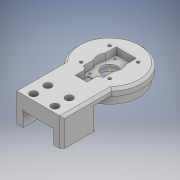
# Autodesk Inventor part: base_top
Saved by Autodesk Inventor 2017 (Build 210142000, 142)
## iProperties
Created: 2021-02-25
Part Number: base_top
Material: Generic
Document SubType Name: Modeling
Designer: paulg
Density: 1 g/cm^3
Appearance: Default
Author: paulg
Autodesk Inventor part; units mm, degrees
ref_plane "YZ Plane" through (0, 0, 0) normal (1, 0, 0) x (0, 1, 0)
ref_plane "XZ Plane" through (0, 0, 0) normal (0, 1, 0) x (-1, 0, 0)
ref_plane "XY Plane" through (0, 0, 0) normal (0, 0, 1) x (1, 0, 0)
sketch "Sketch1" plane through (0, 0, 0) normal (0, 0, 1) x (1, 0, 0)
  circle A0 centre (0, 0) radius 6.5
  circle A1 centre (0, 0) radius 25
  dimension "d0" = 50
  dimension "d1" = 13
  constraints: 2 centre point, 2 coincident
  measures "d0" diameter of A1
  measures "d1" diameter of A0
extrude "Extrusion1" add sketch "Sketch1" along normal blind 7
sketch "Sketch2" plane through (0, 0, 7) normal (0, 0, 1) x (1, 0, 0)
  circle A0 centre (0, 0) radius 6.5 projected
  circle A1 centre (0, 0) radius 25 projected
  circle A2 centre (0, 0) radius 27
  dimension "d4" = 2
  constraints: 1 centre point
  measures "d4" radial gap between concentric circles of A1 A2
extrude "Extrusion2" add sketch "Sketch2" along normal blind 1 contours A1 | A2
sketch "Sketch3" plane through (0, 0, 8) normal (0, 0, 1) x (1, 0, 0)
  circle A0 centre (0, 0) radius 6.5 projected
  circle A1 centre (0, 0) radius 27 projected
  line L0 (0, 0) -> (0, -39.0692) construction
  circle A2 centre (0, 0) radius 27 projected
  line L1 (20, -60) -> (-20, -60)
  line L2 (-20, -60) -> (-20, -18.1384)
  line L3 (-20, -18.1384) -> (20, -18.1384) construction
  line L4 (20, -18.1384) -> (20, -60)
  line L5 (20, -60) -> (-20, -18.1384) construction
  line L6 (-20, -60) -> (20, -18.1384) construction
  arc A3 (-20, -18.1384) -> (20, -18.1384) centre (0, 0) ccw
  dimension "d7" = 40
  dimension "d8" = 60
  constraints: 14 end point, 2 midpoint, 2 parallel, 2 point on circle, 1 centre point, 1 coincident, 1 horizontal, 1 perpendicular, 1 vertical, 4 other
  measures "d7" distance of L1.start L1.end
  measures "d8" distance from line of L1 point (0, 0)
extrude "Extrusion3" add sketch "Sketch3" along normal blind 5
sketch "Sketch4" plane through (0, 0, 0) normal (0, 0, -1) x (-1, 0, 0)
  circle A0 centre (0, 0) radius 6.5 projected
  circle A1 centre (0, 0) radius 25 projected
  line L0 (15.5, -15.5) -> (-15.5, -15.5) construction
  line L1 (-15.5, -15.5) -> (-15.5, 15.5) construction
  line L2 (-15.5, 15.5) -> (15.5, 15.5) construction
  line L3 (15.5, 15.5) -> (15.5, -15.5) construction
  line L4 (15.5, -15.5) -> (-15.5, 15.5) construction
  line L5 (-15.5, -15.5) -> (15.5, 15.5) construction
  dimension "d11" = 31
  constraints: 12 end point, 4 coincident, 2 midpoint, 2 parallel, 2 perpendicular, 1 horizontal
  measures "d11" distance of L2.end L0.start
hole "Hole1" [suppressed]
fillet "Fillet1" [suppressed]
sketch "Sketch5" plane through (0, 0, 0) normal (0, 0, -1) x (-1, 0, 0)
  circle A0 centre (0, 0) radius 25 projected
  circle A1 centre (0, 0) radius 6.5 projected
  line L0 (0, 0) -> (0, 21) construction
  circle A2 centre (0, 0) radius 21 construction
  line L1 (0, 0) -> (8.0364, 19.4015) construction
  point P0 (-8.0364, 19.4015)
  point P1 (-19.4015, 8.0364)
  point P2 (-19.4015, -8.0364)
  point P3 (-8.0364, -19.4015)
  point P4 (8.0364, -19.4015)
  point P5 (19.4015, -8.0364)
  point P6 (19.4015, 8.0364)
  dimension "d20" = 22.5
  dimension "d23" = 360
  dimension "d25" = 42
  constraints: 4 end point, 2 coincident, 2 point on circle, 1 centre point, 1 vertical, 9 other
  measures "d20" angle of L1 L0
  measures "d25" diameter of A2
hole "Hole2" at (-8.0364, 19.4015, 0) at (8.0364, 19.4015, 0) at (19.4015, 8.0364, 0) at (19.4015, -8.0364, 0) at (8.0364, -19.4015, 0) at (-8.0364, -19.4015, 0) at (-19.4015, -8.0364, 0) at (-19.4015, 8.0364, 0) direction (0, 0, 1) diameter 3.2 depth 6 tip angle 118
sketch "Sketch6" plane through (0, 0, 0) normal (0, 0, -1) x (-1, 0, 0)
  circle A0 centre (0, 0) radius 7.5
  dimension "d33" = 15
  constraints: 1 centre point, 1 coincident
  measures "d33" diameter of A0
extrude "Extrusion4" cut sketch "Sketch6" against normal blind 5
sketch "Sketch7" plane through (0, 0, 13) normal (0, 0, 1) x (1, 0, 0)
  line L0 (-8.5, -14) -> (8.5, -14)
  line L1 (8.5, -14) -> (8.5, 14)
  line L2 (8.5, 14) -> (-8.5, 14)
  line L3 (-8.5, 14) -> (-8.5, -14)
  line L4 (-8.5, -14) -> (8.5, 14) construction
  line L5 (8.5, -14) -> (-8.5, 14) construction
  point P0 (0, 0)
  dimension "d36" = 28
  dimension "d37" = 17
  constraints: 12 end point, 2 midpoint, 2 parallel, 1 horizontal, 1 perpendicular
  measures "d36" distance of L0.end L1.end
  measures "d37" distance of L1.end L2.end
extrude "Extrusion5" cut sketch "Sketch7" against normal blind 6
sketch "Sketch8" plane through (0, 0, 0) normal (0, 0, -1) x (-1, 0, 0)
  circle A0 centre (0, 0) radius 10
  dimension "d40" = 20
  constraints: 1 centre point, 1 coincident
  measures "d40" diameter of A0
extrude "Extrusion6" cut sketch "Sketch8" against normal blind 1
sketch "Sketch10" plane through (0, 0, 8) normal (0, 0, -1) x (-1, 0, 0)
  arc A0 (-20, -18.1384) -> (20, -18.1384) centre (0, 0) ccw projected
  line L0 (-20, -18.1384) -> (-20, -60) projected
  line L1 (-20, -60) -> (20, -60) projected
  line L2 (20, -60) -> (20, -18.1384) projected
  circle A1 centre (0, 0) radius 6.5 projected
  arc A2 (-20, -29.9333) -> (20, -29.9333) centre (0, 0) ccw
  dimension "d46" = 36
  constraints: 2 point on circle, 2 point on line, 1 centre point, 1 coincident
  measures "d46" radius of A2
extrude "Extrusion8" add sketch "Sketch10" along normal blind 19 contours A2 L2 L1 L0
sketch "Sketch11" plane through (-20, -60, 13) normal (0, -1, 0) x (1, 0, 0)
  line L0 (40, -24) -> (40, 0) projected
  line L1 (0, 0) -> (40, 0) projected
  line L2 (0, 0) -> (0, -24) projected
  line L3 (40, -24) -> (0, -24) projected
  line L4 (40, -24) -> (0, -24) projected
  line L5 (20, -24) -> (20, -24.5)
  line L6 (32.8, -37.2) -> (7.2, -37.2)
  line L7 (7.2, -37.2) -> (7.2, -11.8)
  line L8 (7.2, -11.8) -> (32.8, -11.8)
  line L9 (32.8, -11.8) -> (32.8, -37.2)
  line L10 (32.8, -37.2) -> (7.2, -11.8) construction
  line L11 (7.2, -37.2) -> (32.8, -11.8) construction
  line L12 (7.2, -12.5071) -> (7.9071, -11.8)
  line L13 (7.9071, -11.8) -> (7.2, -11.0929)
  line L14 (7.2, -11.0929) -> (6.4929, -11.8)
  line L15 (6.4929, -11.8) -> (7.2, -12.5071)
  line L16 (7.2, -12.5071) -> (7.2, -11.0929) construction
  line L17 (7.9071, -11.8) -> (6.4929, -11.8) construction
  line L18 (32.7972, -12.5071) -> (32.0929, -11.7972)
  line L19 (32.0929, -11.7972) -> (32.8028, -11.0929)
  line L20 (32.8028, -11.0929) -> (33.5071, -11.8028)
  line L21 (33.5071, -11.8028) -> (32.7972, -12.5071)
  line L22 (32.7972, -12.5071) -> (32.8028, -11.0929) construction
  line L23 (32.0929, -11.7972) -> (33.5071, -11.8028) construction
  point P0 (20, -13)
  dimension "d49" = 25.6
  dimension "d50" = 25.4
  dimension "d51" = 0.5
  dimension "d52" = 1
  constraints: 38 end point, 7 midpoint, 6 parallel, 4 perpendicular, 3 equal length, 2 horizontal, 1 vertical
  measures "d49" distance of L7.end L8.end
  measures "d50" distance of L8.end L6.start
  measures "d51" distance of L5.start L5.end
  measures "d52" distance of L13.end L14.end
extrude "Extrusion9" cut sketch "Sketch11" against normal blind 22 contours L9 L6 L7 L3 | L3 L7 L12 L8 L18 L21 L9 | L21 L18 L8 L9 | L9 L8 L18 L19 L20 L21 | L15 L14 L13 L8 L7 | L7 L8 L12
fillet "Fillet2" radius 2 2 edges at (20, -29.9333, -1.5) (-20, -29.9333, -1.5)
chamfer "Chamfer1" distance 2 angle 45 5 edges at (20, -39.0692, 13) (-20, -39.0692, 13) (0, 27, 13) (20, -60, 1) (-20, -60, 1)
sketch "Sketch12" plane through (0, 0, 13) normal (0, 0, 1) x (1, 0, 0)
  line L0 (12.0956, -60) -> (12.0956, -38) projected
  line L1 (-12.0929, -60) -> (12.0956, -60) projected
  line L2 (-12.0929, -38) -> (-12.0929, -60) projected
  line L3 (-12.0929, -38) -> (12.0956, -38) projected
  line L4 (-12.0929, -60) -> (12.0956, -60) projected
  line L5 (0.0014, -60) -> (0, 0)
  line L6 (9.0011, -43) -> (-8.9989, -43)
  line L7 (-8.9989, -43) -> (-8.9989, -55)
  line L8 (-8.9989, -55) -> (9.0011, -55)
  line L9 (9.0011, -55) -> (9.0011, -43)
  line L10 (9.0011, -43) -> (-8.9989, -55) construction
  line L11 (-8.9989, -43) -> (9.0011, -55) construction
  point P0 (0.0011, -49)
  dimension "d59" = 5
  dimension "d60" = 5
  dimension "d61" = 18
  constraints: 14 end point, 4 coincident, 3 midpoint, 2 parallel, 1 horizontal, 1 perpendicular, 1 point on line
  measures "d59" distance between parallel lines of L8 L1
  measures "d60" distance between parallel lines of L3 L6
  measures "d61" distance of L7.end L8.end
hole "Hole3" at (-8.9989, -55, 13) at (-8.9989, -43, 13) at (9.0011, -43, 13) at (9.0011, -55, 13) direction (0, 0, -1) diameter 3.2 end through all counterbore diameter 6.2 counterbore depth 7
chamfer "Chamfer2" distance 1.5 angle 45 4 edges at (-8.9989, -39.9, 6) (-8.9989, -51.9, 6) (9.0011, -51.9, 6) (9.0011, -39.9, 6)
sketch "Sketch13" plane through (0, 0, 7) normal (0, 0, 1) x (1, 0, 0)
  line L0 (6, 10.5) -> (-6, 10.5) construction
  line L1 (-6, 10.5) -> (-6, -10.5) construction
  line L2 (-6, -10.5) -> (6, -10.5) construction
  line L3 (6, -10.5) -> (6, 10.5) construction
  line L4 (6, 10.5) -> (-6, -10.5) construction
  line L5 (-6, 10.5) -> (6, -10.5) construction
  point P0 (0, 0)
  dimension "d72" = 12
  dimension "d73" = 21
  constraints: 12 end point, 4 coincident, 2 midpoint, 2 parallel, 1 horizontal, 1 perpendicular
  measures "d72" distance of L0.start L0.end
  measures "d73" distance of L0.end L1.end
hole "Hole4" at (-6, -10.5, 7) at (6, -10.5, 7) at (-6, 10.5, 7) at (6, 10.5, 7) direction (0, 0, -1) diameter 1.5 depth 6 tip angle 90
sketch "Sketch14" plane through (0, 0, 13) normal (0, 0, 1) x (1, 0, 0)
  line L0 (0, 0) -> (0, -69.4768)
  line L1 (5, -19) -> (-5, -19)
  line L2 (-5, -19) -> (-5, -13)
  line L3 (-5, -13) -> (5, -13)
  line L4 (5, -13) -> (5, -19)
  line L5 (5, -19) -> (-5, -13) construction
  line L6 (-5, -19) -> (5, -13) construction
  line L7 (8.5, -14) -> (-8.5, -14) projected
  point P0 (0, -16)
  dimension "d81" = 10
  dimension "d82" = 1
  dimension "d83" = 5
  constraints: 14 end point, 2 midpoint, 2 parallel, 1 horizontal, 1 perpendicular, 1 point on line, 1 vertical
  measures "d81" distance of L1.start L1.end
  measures "d82" distance between parallel lines of L3 L7
  measures "d83" distance between parallel lines of L1 L7
extrude "Extrusion10" cut sketch "Sketch14" against normal blind 7
chamfer "Chamfer3" distance 5 angle 45 1 edges at (0, -19, 13)
chamfer "Chamfer4" distance 2 angle 45 2 edges at (-5, -14, 10) (5, -14, 10)
sketch "Sketch16" plane through (0, 0, 13) normal (0, 0, 1) x (1, 0, 0)
  line L0 (-12, 12) -> (12, 12)
  line L1 (12, 12) -> (12, -12)
  line L2 (12, -12) -> (-12, -12)
  line L3 (-12, -12) -> (-12, 12)
  circle A0 centre (0, 0) radius 10 projected
  line L4 (-12, 12) -> (12, -12) construction
  line L5 (12, 12) -> (-12, -12) construction
  dimension "d92" = 24
  dimension "d93" = 24
  constraints: 12 end point, 4 coincident, 2 midpoint, 2 parallel, 1 horizontal, 1 perpendicular
  measures "d92" distance of L0.start L0.end
  measures "d93" distance of L2.end L0.start
hole "Hole5" at (-12, -12, 13) at (-12, 12, 13) at (12, -12, 13) at (12, 12, 13) direction (0, 0, -1) diameter 2.5 depth 6 tip angle 90
sketch "Sketch17" plane through (0, 0, 13) normal (0, 0, 1) x (1, 0, 0)
  circle A0 centre (12, -12) radius 1.25 projected
  circle A1 centre (-12, -12) radius 1.25 projected
  circle A2 centre (-12, 12) radius 1.25 projected
  circle A3 centre (12, 12) radius 1.25 projected
  circle A4 centre (9.0011, -43) radius 3.1 projected
  circle A5 centre (-8.9989, -55) radius 3.1 projected
  circle A6 centre (-8.9989, -43) radius 3.1 projected
  circle A7 centre (9.0011, -55) radius 3.1 projected
  line L0 (-18, -60) -> (-18, -17.3494) projected
  line L1 (-18, -60) -> (18, -60) projected
  line L2 (18, -17.3494) -> (18, -60) projected
  arc A8 (18, -17.3494) -> (-18, -17.3494) centre (0, 0) ccw projected
  line L3 (5, -16) -> (7, -14) projected
  line L4 (5, -16) -> (5, -24) projected
  line L5 (-5, -24) -> (5, -24) projected
  line L6 (-5, -24) -> (-5, -16) projected
  line L7 (-7, -14) -> (-5, -16) projected
  line L8 (-7, -14) -> (-8.5, -14) projected
  line L9 (-8.5, -14) -> (-8.5, 14) projected
  line L10 (-8.5, 14) -> (8.5, 14) projected
  line L11 (8.5, 14) -> (8.5, -14) projected
  line L12 (8.5, -14) -> (7, -14) projected
  circle A9 centre (0, 0) radius 10
  dimension "d101" = 20
  constraints: 1 centre point, 1 coincident
  measures "d101" diameter of A9
extrude "Extrusion11" cut sketch "Sketch17" against normal up to surface (6 mm away) contours A9 L9 L11 | L11 A9 | A9 L9
sketch "Sketch18" plane through (0, 0, 7) normal (0, 0, 1) x (1, 0, 0)
  point P0 (0, 0)
body "Solid1"
